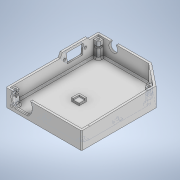
# Autodesk Inventor part: Box_new
Saved by Autodesk Inventor 2020 (Build 240168000, 168)
## iProperties
Created: 2020-04-03
Part Number: Box_new
Material: Generisch
Document SubType Name: Modeling
Designer: Windooof
Density: 1 g/cm^3
Appearance: Vorgabe
Author: Windooof
Autodesk Inventor part; units mm, degrees
ref_plane "YZ Plane" through (0, 0, 0) normal (1, 0, 0) x (0, 1, 0)
ref_plane "XZ Plane" through (0, 0, 0) normal (0, 1, 0) x (-1, 0, 0)
ref_plane "XY Plane" through (0, 0, 0) normal (0, 0, 1) x (1, 0, 0)
sketch "SketchBase" plane through (0, 0, 0) normal (0, 1, 0) x (-1, 0, 0)
  line L0 (45, 55) -> (-45, 55)
  line L1 (-45, 55) -> (-45, -33.701562)
  line L2 (-18.376953, -55) -> (45, -55)
  line L3 (45, -55) -> (45, 55)
  line L4 (63, 0) -> (-63, 0)
  line L5 (0, -77) -> (0, 77)
  line L6 (42.5, 52.5) -> (-42.5, 52.5)
  line L7 (-42.5, 52.5) -> (-42.5, -32.5)
  line L8 (-17.5, -52.5) -> (42.5, -52.5)
  line L9 (42.5, -52.5) -> (42.5, 52.5)
  line L10 (-42.5, 49.5) -> (7.5, 49.5)
  line L11 (7.5, 49.5) -> (7.5, 5.5)
  line L12 (7.5, 5.5) -> (-42.5, 5.5)
  line L13 (-42.5, 5.5) -> (-42.5, 49.5)
  line L14 (-42.5, 49.5) -> (-36.5, 49.5)
  line L15 (-36.5, 49.5) -> (-36.5, 43.5)
  line L16 (-36.5, 43.5) -> (-42.5, 43.5)
  line L17 (-42.5, 43.5) -> (-42.5, 49.5)
  line L18 (7.5, 5.5) -> (0.5, 5.5)
  line L19 (0.5, 5.5) -> (0.5, 12.5)
  line L20 (0.5, 12.5) -> (7.5, 12.5)
  line L21 (7.5, 12.5) -> (7.5, 5.5)
  line L22 (7.5, 49.5) -> (2.5, 49.5)
  line L23 (2.5, 49.5) -> (2.5, 44.5)
  line L24 (2.5, 44.5) -> (7.5, 44.5)
  line L25 (7.5, 44.5) -> (7.5, 49.5)
  line L26 (-42.5, 5.5) -> (-37.5, 5.5)
  line L27 (-37.5, 5.5) -> (-37.5, 10.5)
  line L28 (-37.5, 10.5) -> (-42.5, 10.5)
  line L29 (-42.5, 10.5) -> (-42.5, 5.5)
  line L30 (-42.5, 5.5) -> (-37.5, 5.5)
  line L31 (-37.5, 5.5) -> (-37.5, 3.5)
  line L32 (-37.5, 3.5) -> (-42.5, 3.5)
  line L33 (-42.5, 3.5) -> (-42.5, 5.5)
  line L34 (7.5, 44.5) -> (9.5, 44.5)
  line L35 (9.5, 44.5) -> (9.5, 49.5)
  line L36 (7.5, 49.5) -> (7.5, 44.5)
  line L37 (0.5, 5.5) -> (7.5, 5.5)
  line L38 (7.5, 5.5) -> (7.5, 12.5)
  line L39 (7.5, 12.5) -> (9.5, 12.5)
  line L40 (9.5, 12.5) -> (9.5, 3.5)
  line L41 (9.5, 3.5) -> (0.5, 3.5)
  line L42 (0.5, 3.5) -> (0.5, 5.5)
  line L43 (-36.5, 49.5) -> (-42.5, 49.5)
  line L44 (-42.5, 49.5) -> (-42.5, 52.5)
  line L45 (-42.5, 52.5) -> (-36.5, 52.5)
  line L46 (-36.5, 52.5) -> (-36.5, 49.5)
  line L47 (2.5, 49.5) -> (2.5, 52.5)
  line L48 (2.5, 52.5) -> (9.5, 52.5)
  line L49 (9.5, 52.5) -> (9.5, 49.5)
  line L50 (-17.5, -52.5) -> (-42.5, -32.5)
  line L51 (-45, -33.701562) -> (-18.376953, -55)
  point P0 (0, 0)
  point P1 (-45, -55)
  point P2 (-42.5, -52.5)
  dimension "d0" = 110
  dimension "d1" = 90
  dimension "d2" = 2.5
  dimension "d3" = 2.5
  dimension "d24" = 44
  dimension "d25" = 50
  dimension "d26" = 6
  dimension "d27" = 6
  dimension "d28" = 7
  dimension "d29" = 7
  dimension "d30" = 5
  dimension "d31" = 5
  dimension "d32" = 5
  dimension "d33" = 5
  dimension "d34" = 2
  dimension "d35" = 2
  dimension "d36" = 0
  dimension "d37" = 3
  dimension "d72" = 25
  dimension "d73" = 20
  dimension "d76" = 2.5
  constraints: 100 end point, 20 parallel, 13 perpendicular, 11 horizontal, 6 collinear, 5 point on line, 4 other
  measures "d0" distance of L2.end L0.start
  measures "d1" distance of L0.start L0.end
  measures "d2" distance between parallel lines of L0 L6
  measures "d3" distance between parallel lines of L3 L9
  measures "d24" distance of L11.start L18.start
  measures "d25" distance of L18.start L12.end
  measures "d26" distance of L14.end L15.end
  measures "d27" distance of L15.end L16.end
  measures "d28" distance of L20.start L20.end
  measures "d29" distance of L19.start L20.start
  measures "d30" distance of L24.start L24.end
  measures "d31" distance of L23.start L24.start
  measures "d32" distance of L27.start L27.end
  measures "d33" distance of L27.end L28.end
  measures "d34" distance between parallel lines of L41 L37
  measures "d35" distance between parallel lines of L11 L40
  measures "d36" distance between parallel lines of L7 L13
  measures "d37" distance between parallel lines of L6 L10
  measures "d72" distance of L8.start point (-42.5, -52.5)
  measures "d73" distance of L7.end point (-42.5, -52.5)
  measures "d76" distance between parallel lines of L50 L51
extrude "Base" add sketch "SketchBase" against normal blind 2.5
extrude "Walls" add sketch "SketchBase" along normal blind 23 contours L3 L4 L9 L6 L5 L0 | L5 L6 L7 L4 L1 L0 | L3 L2 L5 L8 L9 L4 | L4 L7 L50 L8 L5 L2 L51 L1
extrude "PCB-Spacer" add sketch "SketchBase" along normal blind 2.5 contours L15 L16 L7 L10 | L10 L11 L24 L23 | L19 L20 L11 L12 | L12 L7 L28 L27
extrude "PCB-Holder" add sketch "SketchBase" along normal blind 4 contours L6 L49 L35 L34 L11 L10 L47 | L46 L10 L7 L6 | L7 L12 L31 L32 | L12 L11 L39 L40 L41 L42
sketch "SketchMounts" plane through (0, 0, 0) normal (0, 1, 0) x (1, 0, 0)
  line L0 (-42.5, 52.5) -> (-36.5, 52.5)
  line L1 (-36.5, 52.5) -> (-36.5, 46.5)
  line L2 (-36.5, 46.5) -> (-42.5, 46.5)
  line L3 (-42.5, 46.5) -> (-42.5, 52.5)
  line L4 (42.5, 32.5) -> (42.5, 25.843142)
  line L5 (42.5, 25.843142) -> (36.232693, 29.487776)
  line L6 (36.232693, 29.487776) -> (37.301867, 36.658506)
  line L7 (37.301867, 36.658506) -> (42.5, 32.5)
  line L8 (-36.5, 52.5) -> (-42.5, 46.5) construction
  line L9 (-36.5, 46.5) -> (-42.5, 52.5) construction
  circle A0 centre (-39.5, 49.5) radius 1.5
  line L10 (42.5, 32.5) -> (36.232693, 29.487776) construction
  circle A1 centre (39.5, 31.058125) radius 1.5
  line L11 (-42.5, -52.5) -> (-36.5, -52.5)
  line L12 (-36.5, -52.5) -> (-36.5, -46.5)
  line L13 (-36.5, -46.5) -> (-42.5, -46.5)
  line L14 (-42.5, -46.5) -> (-42.5, -52.5)
  line L15 (-42.5, -52.5) -> (-36.5, -46.5) construction
  line L16 (-42.5, -46.5) -> (-36.5, -52.5) construction
  circle A2 centre (-39.5, -49.5) radius 1.5
  line L17 (-42.5, -52.5) -> (-42.5, 52.5)
  line L18 (42.5, -52.5) -> (-42.5, -52.5)
  line L19 (-42.5, 52.5) -> (17.5, 52.5)
  line L20 (17.5, 52.5) -> (42.5, 32.5)
  line L21 (42.5, 32.5) -> (42.5, -52.5)
  dimension "d142" = 6
  dimension "d143" = 6
  dimension "d144" = 7.25
  dimension "d145" = 7.25
  dimension "d146" = 3
  dimension "d147" = 3
  dimension "d148" = 6
  dimension "d149" = 3
  dimension "d150" = 6
  dimension "d152" = 3
  dimension "d153" = 3
  constraints: 34 end point, 6 collinear, 4 parallel, 3 centre point, 3 midpoint, 3 perpendicular, 2 horizontal, 2 point on line, 1 other
  measures "d142" distance of L1.start L1.end
  measures "d143" distance of L1.end L2.end
  measures "d144" distance of L6.start L6.end
  measures "d145" distance of L5.start L6.start
  measures "d146" diameter of A0
  measures "d147" diameter of A1
  measures "d148" distance of L12.start L13.start
  measures "d149" diameter of A2
  measures "d150" distance of L13.start L13.end
  measures "d152" distance from line of L6 A1.centre
  measures "d153" distance from line of L7 A1.centre
extrude "Mount1" add sketch "SketchMounts" along normal blind 18 contours L0 L1 L2 L3
extrude "Mount2" add sketch "SketchMounts" along normal blind 18 contours L7 L4 L5 L6
extrude "Mount3" add sketch "SketchMounts" along normal blind 16 contours L13 L12 L11 L14
fillet "RoundingMounts" radius 2 3 edges at (-36.5, 8, 46.5) (-36.5, 9, -46.5) (36.2327, 9, -29.4878)
ref_plane "NutsHeight" through (0, 13, 0) normal (0, 1, 0) x (1, 0, 0)
sketch "SketchNuts" plane through (0, 0, 0) normal (0, 1, 0) x (1, 0, 0)
  circle A0 centre (-39.5, -49.5) radius 1.5
  line L0 (-38.603425, -46.153935) -> (-36.153935, -48.603425)
  line L1 (-36.153935, -48.603425) -> (-37.05051, -51.94949)
  line L2 (-37.05051, -51.94949) -> (-40.396575, -52.846065)
  line L3 (-40.396575, -52.846065) -> (-42.846065, -50.396575)
  line L4 (-42.846065, -50.396575) -> (-41.94949, -47.05051)
  line L5 (-41.94949, -47.05051) -> (-38.603425, -46.153935)
  line L6 (-41.94949, -47.05051) -> (-38.415277, -43.516297)
  line L7 (-38.415277, -43.516297) -> (-33.516297, -48.415277)
  line L8 (-33.516297, -48.415277) -> (-37.05051, -51.94949)
  line L9 (-42.5, -52.5) -> (-35.965787, -45.965787) construction
  circle A1 centre (-39.5, 49.5) radius 1.5
  line L10 (-36.153935, 48.603425) -> (-38.603425, 46.153935)
  line L11 (-38.603425, 46.153935) -> (-41.94949, 47.05051)
  line L12 (-41.94949, 47.05051) -> (-42.846065, 50.396575)
  line L13 (-42.846065, 50.396575) -> (-40.396575, 52.846065)
  line L14 (-40.396575, 52.846065) -> (-37.05051, 51.94949)
  line L15 (-37.05051, 51.94949) -> (-36.153935, 48.603425)
  line L16 (-42.5, -52.5) -> (-42.5, 52.5)
  line L17 (-42.5, 52.5) -> (-34.081244, 44.081244) construction
  line L18 (-41.94949, 47.05051) -> (-36.530733, 41.631754)
  line L19 (-36.530733, 41.631754) -> (-31.631754, 46.530733)
  line L20 (-31.631754, 46.530733) -> (-37.05051, 51.94949)
  circle A2 centre (39.5, 31.058125) radius 1.5
  line L21 (36.045785, 31.319662) -> (37.99939, 34.180331)
  line L22 (37.99939, 34.180331) -> (41.453605, 33.918795)
  line L23 (41.453605, 33.918795) -> (42.954215, 30.796589)
  line L24 (42.954215, 30.796589) -> (41.00061, 27.935919)
  line L25 (41.00061, 27.935919) -> (37.546395, 28.197456)
  line L26 (37.546395, 28.197456) -> (36.045785, 31.319662)
  line L27 (17.5, 52.5) -> (42.5, 32.5)
  line L28 (42.5, 32.5) -> (32.091147, 27.497246) construction
  line L29 (41.00061, 27.935919) -> (33.591756, 24.37504)
  line L30 (33.591756, 24.37504) -> (30.590537, 30.619452)
  line L31 (30.590537, 30.619452) -> (37.99939, 34.180331)
  point P0 (0, 0)
  point P1 (-37.37868, -47.37868)
  point P2 (-41.62132, -51.62132)
  point P3 (-41.62132, 51.62132)
  point P4 (-37.37868, 47.37868)
  point P5 (36.79609, 29.758559)
  point P6 (42.20391, 32.357692)
  point P7 (41.907819, 32.973744)
  point P8 (40.650497, 33.979602)
  point P9 (-42.5, 50.742641)
  point P10 (-42.5, 49.105043)
  point P11 (-42.5, -49.105043)
  point P12 (-42.5, -50.742641)
  dimension "d164" = 6
  dimension "d166" = 6
  dimension "d167" = 6
  constraints: 60 end point, 9 midpoint, 6 perpendicular, 6 point on line, 3 coincident, 2 parallel, 39 other
  measures "d164" distance between parallel lines of L0 L3
  measures "d166" distance between parallel lines of L12 L15
  measures "d167" distance between parallel lines of L24 L21
extrude "Nuts" cut sketch "SketchNuts" against normal blind 2.5 from surface at 13 contours L5 L6 L7 L8 L1 L0 | L0 L1 L2 L3 L16 L4 L5 | L15 L20 L19 L18 L11 L10 | L10 L11 L12 L16 L13 L14 L15 | L26 L25 L29 L30 L31 L21 | L21 L22 L27 L23 L24 L25 L26
chamfer "ChamferBase" distance 2 angle 45 16 edges at (-42.5, 0, 0) (-37.0858, 0, 47.0858) (-40.5, 0, 46.5) (-36.5, 0, 50.5) (-23, 0, 52.5) (17, 0, 52.5) (-9.5, 0, -52.5) (27.4009, 0, -44.5793) (36.8673, 0, -33.7441) (36.6083, 0, -29.6683) (39.9527, 0, -27.3245) (42.5, 0, -11.1716) (42.5, 0, 27) (-37.0858, 0, -47.0858) (-36.5, 0, -50.5) (-40.5, 0, -46.5)
sketch "Skizze3" plane through (-45, 0, 55) normal (0, 0, 1) x (1, 0, 0)
  line L0 (34, 24.5) -> (3, 24.5)
  line L1 (3, 24.5) -> (3, -1.5)
  line L2 (3, -1.5) -> (34, -1.5)
  line L3 (34, -1.5) -> (34, 24.5)
  circle A0 centre (18.5, 11.5) radius 12
  line L4 (18.5, 11.5) -> (34, 11.5) construction
  line L5 (18.5, 11.5) -> (18.5, -1.5) construction
  circle A1 centre (30.5, 21) radius 1.25
  circle A2 centre (6.5, 2) radius 1.25
  line L6 (0, 23) -> (90, 23)
  line L7 (0, -2.5) -> (0, 23)
  line L8 (25.831439, 21) -> (11.168561, 21)
  line L9 (11.168561, 2) -> (25.831439, 2)
  line L10 (90, -2.5) -> (0, -2.5)
  line L11 (62.5, 0) -> (2.5, 0)
  line L12 (26.25, 0) -> (26.25, 11.5) construction
  line L13 (26.25, 11.5) -> (26.25, 23) construction
  point P0 (45, 0)
  point P1 (0, 0)
  dimension "d42" = 26
  dimension "d43" = 31
  dimension "d45" = 24
  dimension "d46" = 2.5
  dimension "d47" = 2.5
  dimension "d48" = 19
  dimension "d49" = 24
  dimension "d50" = 3.5
  dimension "d51" = 3.5
  dimension "d53" = 3
  constraints: 20 end point, 4 point on circle, 4 point on line, 3 centre point, 3 horizontal, 3 midpoint, 3 parallel, 3 vertical, 1 collinear, 1 perpendicular
  measures "d42" distance of L3.start L3.end
  measures "d43" distance of L3.end L0.end
  measures "d45" diameter of A0
  measures "d46" diameter of A1
  measures "d47" diameter of A2
  measures "d48" vertical distance of A2.centre A1.centre
  measures "d49" horizontal distance of A2.centre A1.centre
  measures "d50" distance from line of L0 A1.centre
  measures "d51" distance from line of L3 A1.centre
  measures "d53" distance between parallel lines of L7 L1
extrude "USB-Cutout" cut sketch "Skizze3" against normal blind 10 contours A0 L9 L8 | A1 | A2
sketch "Skizze4" plane through (-45, 0, -55) normal (-1, 0, 0) x (0, 0, 1)
  line L0 (15, 20.5) -> (46, 20.5)
  line L1 (46, 20.5) -> (46, 8)
  line L2 (46, 8) -> (15, 8)
  line L3 (15, 8) -> (15, 20.5)
  line L4 (30.5, 20.5) -> (30.5, 8) construction
  line L5 (20.5, 20.125) -> (40.5, 20.125)
  line L6 (40.5, 20.125) -> (39.5, 8.375)
  line L7 (39.5, 8.375) -> (21.5, 8.375)
  line L8 (21.5, 8.375) -> (20.5, 20.125)
  line L9 (15.173981, 20.125) -> (15.173981, 20.5) construction
  line L10 (15.821992, 8.375) -> (15.821992, 8) construction
  circle A0 centre (18.005, 14.25) radius 1.55
  circle A1 centre (42.995, 14.25) radius 1.55
  line L11 (46, 14.25) -> (15, 14.25) construction
  line L12 (0, -2.5) -> (0, 23)
  line L13 (0, 23) -> (110, 23)
  point P0 (55, 0)
  point P1 (0, 0)
  dimension "d56" = 31
  dimension "d57" = 12.5
  dimension "d58" = 20
  dimension "d59" = 11.75
  dimension "d60" = 18
  dimension "d61" = 3.1
  dimension "d62" = 24.99
  dimension "d63" = 15
  dimension "d64" = 2.5
  constraints: 24 end point, 5 point on line, 4 midpoint, 4 parallel, 3 perpendicular, 2 centre point, 2 horizontal, 1 equal radius, 2 other
  measures "d56" distance of L3.end L1.start
  measures "d57" distance between parallel lines of L2 L0
  measures "d58" distance of L8.end L5.end
  measures "d59" distance between parallel lines of L7 L5
  measures "d60" distance of L7.start L8.start
  measures "d61" diameter of A0
  measures "d62" distance of A1.centre A0.centre
  measures "d63" distance between parallel lines of L12 L3
  measures "d64" distance between parallel lines of L13 L0
extrude "Stepper-Cutout" cut sketch "Skizze4" against normal blind 2.5 contours L5 L6 L7 L8 | A0 | A1
sketch "Skizze5" plane through (45, 0, -55) normal (0, 0, -1) x (-1, 0, 0)
  circle A0 centre (69.75, 15.25) radius 5.25
  line L0 (90, -2.5) -> (90, 23)
  line L1 (26.623047, 23) -> (90, 23)
  point P0 (45, 0)
  point P1 (90, 0)
  point P2 (0, 28)
  dimension "d67" = 10.5
  dimension "d68" = 20.25
  dimension "d69" = 7.75
  constraints: 1 centre point, 1 other
  measures "d67" diameter of A0
  measures "d68" distance from line of L0 A0.centre
extrude "Power-Cutout" cut sketch "Skizze5" against normal blind 2.5
sketch "Skizze7" plane through (-45, -2.5, 55) normal (0, 0, 1) x (1, 0, 0)
  line L0 (90, 0) -> (90, 25.5)
  line L1 (90, 20.5) -> (28.587121, 20.5)
  arc A0 (8.5, 7.36675) -> (11.168561, 4.5) centre (18.5, 14) ccw
  arc A1 (28.587121, 20.5) -> (25.831439, 23.5) centre (18.5, 14) ccw
  line L2 (25.831439, 23.5) -> (11.168561, 23.5)
  line L3 (25.831439, 23.5) -> (11.168561, 23.5)
  line L4 (8.412879, 20.5) -> (0, 20.5)
  line L5 (0, 0) -> (0, 25.5)
  arc A2 (8.5, 7.36675) -> (11.168561, 4.5) centre (18.5, 14) ccw
  arc A3 (11.168561, 23.5) -> (11.168561, 4.5) centre (18.5, 14) ccw
  line L6 (0, 25.5) -> (90, 25.5)
  arc A4 (11.168561, 23.5) -> (8.412879, 20.5) centre (18.5, 14) ccw
  line L7 (0, 20.5) -> (0, 25.5)
  line L8 (90, 25.5) -> (63.376953, 25.5)
  line L9 (90, 20.5) -> (90, 25.5)
  line L10 (90, 25.5) -> (0, 25.5)
  point P0 (45, 2.5)
  point P1 (25.831439, 4.5)
  dimension "d81" = 5
  constraints: 12 end point, 6 point on circle, 2 centre point, 2 collinear, 2 concentric, 2 horizontal, 2 point on line, 2 vertical, 1 perpendicular
  measures "d81" distance between parallel lines of L6 L1
extrude "TopCutout1" cut sketch "Skizze7" against normal blind 2.5
sketch "Skizze8" plane through (-45, -2.5, -55) normal (-1, 0, 0) x (0, 0, 1)
  line L0 (110, 20.5) -> (48, 20.5)
  line L1 (0, 25.5) -> (107.5, 25.5)
  line L2 (39.5, 10.875) -> (21.5, 10.875)
  line L3 (30.5, 10.875) -> (30.5, 22.625) construction
  line L4 (40.5, 22.625) -> (20.5, 22.625)
  line L5 (0, 25.5) -> (110, 25.5)
  line L6 (110, 25.5) -> (110, 20.5)
  line L7 (13, 22.5) -> (0, 22.5)
  line L8 (13, 29.29359) -> (13, 14.81546) construction
  line L9 (48, 30.210757) -> (48, 14.291365) construction
  line L10 (0, 25.5) -> (0, 22.5)
  line L11 (15.5, 25.5) -> (13, 22.5)
  line L12 (45.5, 25.5) -> (48, 20.5)
  line L13 (15.5, 25.5) -> (45.5, 25.5)
  line L14 (0, 0) -> (0, 25.5)
  point P0 (55, 2.5)
  dimension "d97" = 35
  dimension "d98" = 3
  dimension "d137" = 30
  constraints: 22 end point, 5 point on line, 3 vertical, 2 horizontal, 2 midpoint, 1 collinear, 1 symmetric about line, 1 other
  measures "d97" horizontal distance of L0.end L7.start
  measures "d98" distance between parallel lines of L1 L7
  measures "d137" distance of L11.start L12.start
extrude "TopCutout2" cut sketch "Skizze8" against normal blind 2.5
sketch "Skizze9" plane through (18.376953, -2.5, -55) normal (0, 0, -1) x (-1, 0, 0)
  line L0 (0, 0) -> (0, 25.5)
  line L1 (0, 22.5) -> (0, 25.5)
  line L2 (0, 25.5) -> (63.376953, 25.5)
  line L3 (63.376953, 25.5) -> (63.376953, 22.5)
  line L4 (0, 22.5) -> (40.890885, 22.5)
  circle A0 centre (43.126953, 17.75) radius 5.25
  line L5 (45.363021, 22.5) -> (63.376953, 22.5)
  circle A1 centre (43.126953, 17.75) radius 5.25
  arc A2 (45.363021, 22.5) -> (40.890885, 22.5) centre (43.126953, 17.75) ccw
  constraints: 10 end point, 3 point on circle, 2 point on line, 1 centre point, 1 coincident, 1 collinear, 1 concentric, 1 horizontal, 1 parallel, 2 other
extrude "TopCutout3" cut sketch "Skizze9" against normal blind 2.5 contours L0 L2 L3 L5 A0 L4
sketch "Skizze12" plane through (45, -2.5, -33.701562) normal (0.624695, 0, -0.7808688) x (-0.7808688, 0, -0.624695)
  line L0 (34.094136, 22.5) -> (0, 22.5)
  line L1 (0, 22.5) -> (0, 25.5)
  line L2 (0, 25.5) -> (34.094136, 25.5)
  line L3 (34.094136, 25.5) -> (34.094136, 22.5)
  line L4 (66.024552, 22.5) -> (34.094136, 22.5)
  point P0 (14.085897, 2.5)
  constraints: 8 end point, 2 parallel, 1 collinear, 1 horizontal, 1 perpendicular
extrude "TopCutout4" cut sketch "Skizze12" against normal blind 2.5
sketch "Skizze13" plane through (45, -2.5, 55) normal (1, 0, 0) x (0, 0, -1)
  line L0 (0, 4.5) -> (0, 20.5)
  line L1 (0, 20.5) -> (10, 20.5)
  line L2 (10, 20.5) -> (78.701562, 22.5)
  line L3 (78.701562, 22.5) -> (88.701562, 22.5)
  line L4 (0, 20.5) -> (0, 25.5)
  line L5 (0, 25.5) -> (88.701562, 25.5)
  line L6 (88.701562, 25.5) -> (88.701562, 22.5)
  line L7 (2.5, 20.5) -> (0, 20.5)
  point P0 (55, 2.5)
  dimension "d105" = 10
  dimension "d106" = 10
  constraints: 12 end point, 1 coincident, 1 collinear, 1 horizontal, 1 perpendicular, 1 vertical
  measures "d105" distance of L0.end L1.end
  measures "d106" distance of L3.end L2.end
extrude "TopCutout5" cut sketch "Skizze13" against normal blind 2.5
chamfer "ChamferOutside" distance 1 angle 45 3 edges at (45, 7.75, 55) (-45, 7.75, 55) (-45, 8.75, -55)
fillet "RoundingPower" radius 0.5 2 edges at (-22.5139, 20, -53.75) (-26.9861, 20, -53.75)
fillet "RoundingCutouts" radius 0.75 11 edges at (-38.3259, 9.4632, 55) (-26.5, 2, 55) (-14.6741, 9.4632, 55) (-45, 8.375, -24.5) (-45, 14.25, -34) (-45, 20.125, -24.5) (-45, 14.25, -15) (-43.75, 8.375, -33.5) (-43.75, 8.375, -15.5) (-43.75, 20.125, -14.5) (-43.75, 20.125, -34.5)
